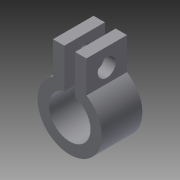
# Autodesk Inventor part: Collar Piece Thingy
Saved by Autodesk Inventor 2014 (Build 180170000, 170)
## iProperties
Created: 2013-08-07
Part Number: Collar Piece Thingy
Material: Generic
Document SubType Name: Modeling
Designer: Nick
Density: 1 g/cm^3
Appearance: Default
Author: Nick
Autodesk Inventor part; units mm, degrees
ref_plane "YZ Plane" through (0, 0, 0) normal (1, 0, 0) x (0, 1, 0)
ref_plane "XZ Plane" through (0, 0, 0) normal (0, 1, 0) x (-1, 0, 0)
ref_plane "XY Plane" through (0, 0, 0) normal (0, 0, 1) x (1, 0, 0)
sketch "Sketch1" plane through (0, 0, 0) normal (0, 0, 1) x (1, 0, 0)
  arc A0 (-0.9525, 3.5494) -> (0.9525, 3.5494) centre (0, 0) ccw
  arc A1 (-2.9525, 4.8465) -> (2.9525, 4.8465) centre (0, 0) ccw
  line L0 (-0.9525, 10.525) -> (-0.9525, 3.5494)
  line L1 (0.9525, 3.5494) -> (0.9525, 10.525)
  line L2 (2.9525, 10.525) -> (2.9525, 4.8465)
  line L3 (-2.9525, 10.525) -> (-2.9525, 4.8465)
  line L4 (-2.9525, 10.525) -> (-0.9525, 10.525)
  line L5 (0.9525, 10.525) -> (2.9525, 10.525)
  dimension "d6" = 7.35
  dimension "d12" = 2
  dimension "d13" = 2
  dimension "d14" = 1.905
  dimension "d15" = 0.9525
  dimension "d17" = 10.525
  dimension "d18" = 10.525
  dimension "d32" = 2
  constraints: 12 end point, 4 perpendicular, 4 point on circle, 2 centre point, 2 coincident, 2 parallel, 1 vertical
  measures "d6" diameter of A0
  measures "d12" distance between parallel lines of L0 L3
  measures "d13" distance between parallel lines of L2 L1
  measures "d14" distance between parallel lines of L1 L0
  measures "d15" distance from line of point (0, 0) L0
  measures "d17" distance from line of point (0, 0) L4
  measures "d18" distance from line of point (0, 0) L5
  measures "d32" radial gap between concentric circles of A0 A1
extrude "Extrusion1" add sketch "Sketch1" along normal blind 7.175
sketch "Sketch3" plane through (0, 0, 0) normal (1, 0, 0) x (0, 1, 0)
  circle A0 centre (7.35, 3.5875) radius 1.5875
  line L0 (10.525, 0) -> (10.525, 7.175) projected
  point P0 (0, 0)
  dimension "d25" = 3.175
  dimension "d27" = 3.5875
  dimension "d28" = 7.35
  dimension "d29" = 7.175
  constraints: 1 centre point
  measures "d25" diameter of A0
  measures "d27" vertical distance of point (0, 0) A0.centre
  measures "d28" horizontal distance of point (0, 0) A0.centre
  measures "d29" distance of L0.start L0.end
extrude "Extrusion2" cut sketch "Sketch3" along normal mid plane 5.905
equation "\"d13\" = d12"
equation "\"d15\" = 0.5 * d14"
equation "\"d18\" = d17"
equation "\"d27\" = 0.5 * d29"
equation "\"d30\" = 2 * d12 + 2 * d15"
body "Solid1"
